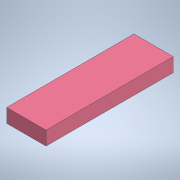
# Autodesk Inventor part: Bateria
Saved by Autodesk Inventor 2022 (Build 260153000, 153)
## iProperties
Created: 2021-08-09
Part Number: Bateria
Material: Ogólny
Document SubType Name: Modeling
Designer: Krystyna
Density: 2.85205 g/cm^3
Appearance: Domyślna
Mass: 16 g
Surface Area: 27.34 cm^2
Volume: 5.61 cm^3
Author: Krystyna
Autodesk Inventor part; units mm, degrees
ref_plane "YZ Plane" through (0, 0, 0) normal (1, 0, 0) x (0, 1, 0)
ref_plane "XZ Plane" through (0, 0, 0) normal (0, 1, 0) x (-1, 0, 0)
ref_plane "XY Plane" through (0, 0, 0) normal (0, 0, 1) x (1, 0, 0)
sketch "Szkic1" plane through (0, 0, 0) normal (0, 1, 0) x (-1, 0, 0)
  line L0 (8.5, 27.5) -> (-8.5, 27.5)
  line L1 (-8.5, 27.5) -> (-8.5, -27.5)
  line L2 (-8.5, -27.5) -> (8.5, -27.5)
  line L3 (8.5, -27.5) -> (8.5, 27.5)
  point P0 (0, 0)
  point P1 (8.5, 0)
  point P2 (0, -27.5)
  dimension "d0" = 55
  dimension "d1" = 17
  constraints: 8 end point, 2 midpoint, 2 parallel, 1 horizontal, 1 horizontal alignment, 1 perpendicular, 1 vertical alignment
  measures "d0" distance of L2.end L0.start
  measures "d1" distance of L1.end L2.end
extrude "Wyciągnięcie proste1" add sketch "Szkic1" along normal blind 6
